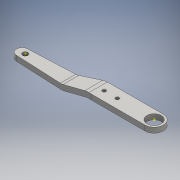
# Autodesk Inventor part: Profile_Straight_03
Saved by Autodesk Inventor 2016 (Build 200138000, 138)
## iProperties
Created: 2016-02-08
Part Number: Profile_Straight_03
Material: Generic
Document SubType Name: Modeling
Designer: nils
Density: 1 g/cm^3
Appearance: Default
Mass: 606.719 g
Surface Area: 940.542 cm^2
Volume: 606.719 cm^3
Author: nils
Autodesk Inventor part; units mm, degrees
ref_plane "YZ Plane" through (0, 0, 0) normal (1, 0, 0) x (0, 1, 0)
ref_plane "XZ Plane" through (0, 0, 0) normal (0, 1, 0) x (-1, 0, 0)
ref_plane "XY Plane" through (0, 0, 0) normal (0, 0, 1) x (1, 0, 0)
sketch "Sketch4" plane through (0, 0, 0) normal (1, 0, 0) x (0, 1, 0)
  line L0 (-35, 10) -> (35, 10)
  line L1 (35, 10) -> (35, -10)
  line L2 (35, -10) -> (-35, -10)
  line L3 (-35, -10) -> (-35, 10)
  line L4 (-35, 10) -> (35, -10) construction
  line L5 (35, 10) -> (-35, -10) construction
  point P0 (0, 0)
  dimension "d15" = 20
  dimension "d16" = 70
  constraints: 12 end point, 2 midpoint, 2 parallel, 1 horizontal, 1 perpendicular
  measures "d15" distance between parallel lines of L2 L0
  measures "d16" distance of L1.end L2.end
sketch "Sketch5" plane through (0, 0, 0) normal (0, 1, 0) x (-1, 0, 0)
  line L0 (0, 0) -> (220, 0)
  line L1 (220, 0) -> (320, -28.8125)
  line L2 (320, -28.8125) -> (490, -28.8125)
  dimension "d17" = 490
  dimension "d18" = 220
  dimension "d19" = 320
  constraints: 6 end point, 1 horizontal, 1 parallel
  measures "d17" horizontal distance of L0.start L2.end
  measures "d18" distance of L0.start L0.end
  measures "d19" horizontal distance of L0.start L1.end
sweep "Sweep1" add profiles "Sketch4" path "Sketch5"
sketch "Sketch9" plane through (0, -35, 10) normal (1, 0, 0) x (0, 0, -1)
  line L0 (0, 0) -> (0, 70) projected
  line L1 (20, 0) -> (0, 0) projected
  line L2 (0, 70) -> (20, 70)
  line L3 (20, 70) -> (20, 0)
  line L4 (20, 0) -> (0, 0)
  line L5 (0, 0) -> (0, 70)
  point P0 (10, 35)
  constraints: 8 end point, 2 parallel, 1 horizontal, 1 perpendicular
extrude "Extrusion2" add sketch "Sketch9" along normal blind 35
sketch "Sketch10" plane through (-490, -35, -18.8125) normal (-1, 0, 0) x (0, 0, 1)
  line L0 (8.8125, 70) -> (-20, 70) projected
  line L1 (0, 0) -> (0, 70) projected
  line L2 (-20, 70) -> (0, 70)
  line L3 (0, 70) -> (0, 0)
  line L4 (0, 0) -> (-20, 0)
  line L5 (-20, 0) -> (-20, 70)
  point P0 (18.8125, 35)
  constraints: 8 end point, 2 parallel, 1 horizontal, 1 perpendicular
extrude "Extrusion3" add sketch "Sketch10" along normal blind 32.5
hole "Hole1" at (0, 0, 10) direction (0, 0, -1) diameter 55 end through all
hole "Hole2" at (-490, 0, -18.8125) direction (0, 0, -1) diameter 20 end through all
sketch "Sketch12" plane through (-318.5881, -35, -38.8125) normal (0, 0, -1) x (-1, 0, 0)
  line L0 (151.4119, 20) -> (191.4119, 20)
  line L1 (191.4119, 20) -> (191.4119, 50)
  line L2 (191.4119, 50) -> (151.4119, 50)
  line L3 (151.4119, 50) -> (151.4119, 20)
  line L4 (151.4119, 20) -> (191.4119, 50) construction
  line L5 (191.4119, 20) -> (151.4119, 50) construction
  line L6 (0, 0) -> (203.9119, 0) projected
  point P0 (-318.5881, 35)
  point P1 (171.4119, 35)
  dimension "d44" = 40
  dimension "d45" = 30
  dimension "d46" = 35
  dimension "d47" = 490
  constraints: 12 end point, 2 midpoint, 2 parallel, 1 horizontal, 1 perpendicular
  measures "d44" distance of L1.end L2.end
  measures "d45" distance of L0.end L1.end
  measures "d46" distance from line of L6 point (171.412, 35)
  measures "d47" distance of point (171.412, 35) point (-318.588, 35)
extrude "Extrusion4" cut sketch "Sketch12" against normal blind 10
fillet "Fillet1" radius 40 2 edges at (-218.5881, 0, -10) (-321.4119, 0, -18.8125)
fillet "Fillet2" radius 60 2 edges at (-221.4119, 0, 10) (-318.5881, 0, -38.8125)
fillet "Fillet3" radius 35 2 edges at (35, 35, 0) (35, -35, 0)
fillet "Fillet4" radius 8 4 edges at (-470, 15, -33.8125) (-510, 15, -33.8125) (-470, -15, -33.8125) (-510, -15, -33.8125)
sketch "Sketch15" plane through (-522.5, -35, -38.8125) normal (0, 0, -1) x (-1, 0, 0)
  line L0 (0, 0) -> (0, 70) projected
  line L1 (0, 55) -> (-320, 70)
  line L2 (-522.5, 70) -> (-309.5595, 70) projected
  line L3 (-195.4405, 70) -> (0, 70) projected
  line L4 (0, 70) -> (-320, 70)
  line L5 (0, 70) -> (0, 55)
  line L6 (0, 15) -> (-320, 0)
  line L7 (-522.5, 0) -> (-309.5595, 0) projected
  line L8 (-195.4405, 0) -> (0, 0) projected
  line L9 (0, 0) -> (0, 15)
  line L10 (-320, 70) -> (-320, 0) construction
  line L11 (-320, 0) -> (0, 0)
  point P0 (-522.5, 35)
  dimension "d73" = 15
  dimension "d74" = 40
  dimension "d75" = 320
  constraints: 14 end point, 4 point on line, 3 collinear, 1 horizontal, 1 perpendicular
  measures "d73" distance from line of L3 L1.start
  measures "d74" distance of L6.start L1.start
  measures "d75" distance between parallel lines of L0 L10
extrude "Extrusion6" cut sketch "Sketch15" against normal through all
fillet "Fillet7" radius 20 2 edges at (-522.5, -20, -28.8125) (-522.5, 20, -28.8125)
sketch "Sketch19" plane through (0, 0, -10) normal (0, 0, -1) x (-1, 0, 0)
  line L0 (0, 0) -> (490, 0)
  point P0 (190, 0)
  point P1 (140, 0)
  dimension "d112" = 140
  dimension "d113" = 190
  constraints: 2 end point, 2 point on line, 1 horizontal
  measures "d112" distance of point (140, 0) L0.start
  measures "d113" distance of L0.start point (190, 0)
hole "Hole6" at (-490, 0, -10) at (-190, 0, -10) at (-140, 0, -10) direction (0, 0, 1) diameter 13.5 end through all countersink diameter 27.2 countersink angle 90
body "Solid2"
